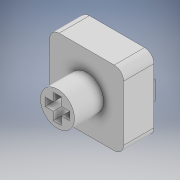
# Autodesk Inventor part: IPC ENTR key
Saved by Autodesk Inventor 2022 (Build 260153000, 153)
## iProperties
Created: 2021-12-31
Part Number: IPC ENTR key
Material: Generic
Document SubType Name: Modeling
Designer: solor
Density: 1 g/cm^3
Appearance: Default
Author: solor
Autodesk Inventor part; units mm, degrees
ref_plane "YZ Plane" through (0, 0, 0) normal (1, 0, 0) x (0, 1, 0)
ref_plane "XZ Plane" through (0, 0, 0) normal (0, 1, 0) x (-1, 0, 0)
sketch "Sketch1" plane through (0, 0, 0) normal (0, 0, 1) x (1, 0, 0)
  line L0 (14.6962, 12.74) -> (14.6962, 0) construction
  line L1 (10.61, 12.2) -> (1.53, 12.2)
  arc A0 (1.53, 12.2) -> (0, 10.67) centre (1.53, 10.67) ccw
  line L2 (0, 10.67) -> (0, 1.53)
  arc A1 (0, 1.53) -> (1.53, 0) centre (1.53, 1.53) ccw
  line L3 (1.53, 0) -> (10.61, 0)
  arc A2 (10.61, 0) -> (12.14, 1.53) centre (10.61, 1.53) ccw
  arc A3 (12.14, 10.67) -> (10.61, 12.2) centre (10.61, 10.67) ccw
  line L4 (12.14, 10.67) -> (12.14, 1.53)
  point P0 (0, 0)
  point P1 (0, 0)
  dimension "d10" = 12.74
  constraints: 10 end point, 8 point on circle, 4 centre point, 2 vertical, 1 point on line
  measures "d10" distance of L0.start L0.end
ref_plane "Work Plane1" through (0, 0, 5) normal (0, 0, 1) x (1, 0, 0)
sketch "Sketch2" plane through (0, 0, 5) normal (0, 0, 1) x (1, 0, 0)
  line L0 (10.88, 12.74) -> (1.8, 12.74) projected
  line L1 (10.88, 12.74) -> (1.8, 12.74) projected
  arc A0 (1.8, 12.74) -> (0, 10.94) centre (1.8, 10.94) ccw projected
  line L2 (0, 10.94) -> (0, 1.8) projected
  arc A1 (0, 1.8) -> (1.8, 0) centre (1.8, 1.8) ccw projected
  line L3 (1.8, 0) -> (10.88, 0) projected
  arc A2 (10.88, 0) -> (12.68, 1.8) centre (10.88, 1.8) ccw projected
  line L4 (12.68, 1.8) -> (12.68, 10.94) projected
  arc A3 (12.68, 10.94) -> (10.88, 12.74) centre (10.88, 10.94) ccw projected
  circle A4 centre (6.34, 6.37) radius 2.8
  line L5 (5.665, 8.395) -> (7.015, 8.395)
  line L6 (7.015, 4.345) -> (5.665, 4.345)
  line L7 (5.665, 4.345) -> (7.015, 8.395) construction
  line L8 (5.665, 8.395) -> (7.015, 4.345) construction
  line L9 (8.365, 5.695) -> (8.365, 7.045)
  line L10 (4.315, 7.045) -> (4.315, 5.695)
  line L11 (4.315, 5.695) -> (8.365, 7.045) construction
  line L12 (8.365, 5.695) -> (4.315, 7.045) construction
  line L13 (4.315, 5.695) -> (5.665, 5.695)
  line L14 (7.015, 5.695) -> (8.365, 5.695)
  line L15 (5.665, 4.345) -> (5.665, 5.695)
  line L16 (5.665, 7.045) -> (5.665, 8.395)
  line L17 (8.365, 7.045) -> (7.015, 7.045)
  line L18 (5.665, 7.045) -> (4.315, 7.045)
  line L19 (7.015, 8.395) -> (7.015, 7.045)
  line L20 (7.015, 5.695) -> (7.015, 4.345)
  point P0 (0, 0)
  dimension "d3" = 5.6
  dimension "d4" = 4.05
  dimension "d5" = 1.35
  dimension "d6" = 4.05
  dimension "d7" = 1.35
  constraints: 32 end point, 10 parallel, 8 perpendicular, 4 midpoint, 2 vertical, 1 centre point
  measures "d3" diameter of A4
  measures "d4" distance of L6.end L5.start
  measures "d5" distance of L5.start L5.end
  measures "d6" distance of L10.end L9.start
  measures "d7" distance of L9.end L9.start
extrude "Extrusion3" add sketch "Sketch1" along normal blind 5
sketch "Sketch3" plane through (0, 0, 5) normal (0, 0, 1) x (1, 0, 0)
  line L0 (10.61, 12.47) -> (1.53, 12.47)
  line L1 (10.61, 12.47) -> (1.53, 12.47)
  arc A0 (1.53, 12.47) -> (-0.27, 10.67) centre (1.53, 10.67) ccw
  line L2 (-0.27, 10.67) -> (-0.27, 1.53)
  arc A1 (-0.27, 1.53) -> (1.53, -0.27) centre (1.53, 1.53) ccw
  line L3 (1.53, -0.27) -> (10.61, -0.27)
  arc A2 (10.61, -0.27) -> (12.41, 1.53) centre (10.61, 1.53) ccw
  line L4 (12.41, 1.53) -> (12.41, 10.67)
  arc A3 (12.41, 10.67) -> (10.61, 12.47) centre (10.61, 10.67) ccw
  circle A4 centre (6.07, 6.1) radius 2.8
  line L5 (5.395, 8.125) -> (6.745, 8.125)
  line L6 (6.745, 4.075) -> (5.395, 4.075)
  line L7 (5.395, 4.075) -> (6.745, 8.125) construction
  line L8 (5.395, 8.125) -> (6.745, 4.075) construction
  line L9 (8.095, 5.425) -> (8.095, 6.775)
  line L10 (4.045, 6.775) -> (4.045, 5.425)
  line L11 (4.045, 5.425) -> (8.095, 6.775) construction
  line L12 (8.095, 5.425) -> (4.045, 6.775) construction
  line L13 (4.045, 5.425) -> (5.395, 5.425)
  line L14 (6.745, 5.425) -> (8.095, 5.425)
  line L15 (5.395, 4.075) -> (5.395, 5.425)
  line L16 (5.395, 6.775) -> (5.395, 8.125)
  line L17 (8.095, 6.775) -> (6.745, 6.775)
  line L18 (5.395, 6.775) -> (4.045, 6.775)
  line L19 (6.745, 8.125) -> (6.745, 6.775)
  line L20 (6.745, 5.425) -> (6.745, 4.075)
  line L21 (10.61, 12.2) -> (1.53, 12.2) projected
  line L22 (0, 10.67) -> (0, 1.53) projected
  point P0 (0, 0)
  point P1 (-0.27, -0.27)
  point P2 (6.07, 12.2)
  point P3 (0, 6.1)
  point P4 (6.07, 6.1)
  dimension "d14" = 5.6
  dimension "d15" = 4.05
  dimension "d16" = 1.35
  dimension "d17" = 4.05
  dimension "d18" = 1.35
  constraints: 42 end point, 10 parallel, 8 perpendicular, 8 point on circle, 6 midpoint, 5 centre point, 2 vertical
  measures "d14" diameter of A4
  measures "d15" distance of L6.end L5.start
  measures "d16" distance of L5.start L5.end
  measures "d17" distance of L10.end L9.start
  measures "d18" distance of L9.end L9.start
extrude "Extrusion4" add sketch "Sketch3" along normal blind 4.8 contours A4
sketch "Sketch4" plane through (0, 0, 0) normal (0, 0, -1) x (-1, 0, 0)
  line L0 (-13.9436, 0) -> (-13.9436, 2.266)
  line L1 (-15.5559, 0) -> (-15.5559, 6.84)
  line L2 (-1.53, 0) -> (-10.61, 0) projected
  line L3 (-11.7832, 7.625) -> (-0.3568, 7.625) construction
  line L4 (-0.3568, 7.625) -> (-0.3568, 4.575) construction
  line L5 (-0.3568, 4.575) -> (-11.7832, 4.575) construction
  line L6 (-11.7832, 4.575) -> (-11.7832, 7.625) construction
  line L7 (-11.4668, 4.575) -> (-11.4668, 7.625)
  line L8 (-11.4668, 7.625) -> (-9.4055, 7.625)
  line L9 (-9.4055, 7.625) -> (-9.4055, 7.0442)
  line L10 (-9.4055, 7.0442) -> (-10.7056, 7.0442)
  line L11 (-10.7056, 7.0442) -> (-10.7056, 6.5078)
  line L12 (-10.7056, 6.5078) -> (-9.5068, 6.5078)
  line L13 (-9.5068, 6.5078) -> (-9.5068, 5.927)
  line L14 (-9.5068, 5.927) -> (-10.7056, 5.927)
  line L15 (-10.7056, 5.927) -> (-10.7056, 5.1558)
  line L16 (-10.7056, 5.1558) -> (-9.4055, 5.1558)
  line L17 (-9.4055, 5.1558) -> (-9.4055, 4.575)
  line L18 (-9.4055, 4.575) -> (-11.4668, 4.575)
  line L19 (-6.2739, 4.575) -> (-7.0105, 4.575)
  line L20 (-7.0105, 4.575) -> (-8.187, 6.7006)
  line L21 (-8.187, 6.7006) -> (-8.187, 4.575)
  line L22 (-8.187, 4.575) -> (-8.8864, 4.575)
  line L23 (-8.8864, 4.575) -> (-8.8864, 7.625)
  line L24 (-8.8864, 7.625) -> (-7.9472, 7.625)
  line L25 (-7.9472, 7.625) -> (-6.9734, 5.8776)
  line L26 (-6.9734, 5.8776) -> (-6.9734, 7.625)
  line L27 (-6.9734, 7.625) -> (-6.2739, 7.625)
  line L28 (-6.2739, 7.625) -> (-6.2739, 4.575)
  line L29 (-5.0678, 4.575) -> (-5.0678, 7.0442)
  line L30 (-5.0678, 7.0442) -> (-5.9699, 7.0442)
  line L31 (-5.9699, 7.0442) -> (-5.9699, 7.625)
  line L32 (-5.9699, 7.625) -> (-3.3994, 7.625)
  line L33 (-3.3994, 7.625) -> (-3.3994, 7.0442)
  line L34 (-3.3994, 7.0442) -> (-4.3015, 7.0442)
  line L35 (-4.3015, 7.0442) -> (-4.3015, 4.575)
  line L36 (-4.3015, 4.575) -> (-5.0678, 4.575)
  line L37 (-0.2678, 4.575) -> (-1.1996, 4.575)
  line L38 (-1.1996, 4.575) -> (-2.0474, 5.6947)
  line L39 (-2.0474, 5.6947) -> (-2.3242, 5.6947)
  line L40 (-2.3242, 5.6947) -> (-2.3242, 4.575)
  line L41 (-2.3242, 4.575) -> (-3.0855, 4.575)
  line L42 (-3.0855, 4.575) -> (-3.0855, 7.625)
  line L43 (-3.0855, 7.625) -> (-1.8596, 7.625)
  spline S0 degree 2 poles (-1.8596, 7.625) (-1.605, 7.625) (-1.2293, 7.5607) (-1.0686, 7.4619) knots 0 0 0 1 2 2 2
  spline S1 degree 2 poles (-1.0686, 7.4619) (-0.9055, 7.3581) (-0.7127, 7.0343) (-0.7127, 6.7871) knots 0 0 0 1 2 2 2
  spline S2 degree 2 poles (-0.7127, 6.7871) (-0.7127, 6.4386) (-1.0291, 6.0011) (-1.2936, 5.8726) knots 0 0 0 1 2 2 2
  line L44 (-1.2936, 5.8726) -> (-0.2678, 4.575)
  spline S3 degree 2 poles (-1.4987, 6.6907) (-1.4987, 6.8069) (-1.5877, 6.9725) (-1.689, 7.017) knots 0 0 0 1 2 2 2
  spline S4 degree 2 poles (-1.689, 7.017) (-1.7607, 7.0466) (-1.9362, 7.0639) (-2.0672, 7.0639) knots 0 0 0 1 2 2 2
  line L45 (-2.0672, 7.0639) -> (-2.3242, 7.0639)
  line L46 (-2.3242, 7.0639) -> (-2.3242, 6.2434)
  line L47 (-2.3242, 6.2434) -> (-2.1043, 6.2434)
  spline S5 degree 2 poles (-2.1043, 6.2434) (-1.9461, 6.2434) (-1.7212, 6.2829) (-1.6445, 6.3447) knots 0 0 0 1 2 2 2
  spline S6 degree 2 poles (-1.6445, 6.3447) (-1.5704, 6.404) (-1.4987, 6.5622) (-1.4987, 6.6907) knots 0 0 0 1 2 2 2
  point P0 (0, 0)
  point P1 (-6.07, 0)
  point P2 (-6.07, 2.266)
  point P3 (-6.07, 6.84)
  point P4 (-6.07, 6.1)
  point P5 (-6.07, 4.575)
  point P6 (-0.3568, 6.1)
  point P7 (-6.07, 6.1)
  dimension "d21" = 2.266
  dimension "d22" = 6.84
  constraints: 4 end point, 3 midpoint, 2 vertical, 2 other
  measures "d21" distance of L0.start L0.end
  measures "d22" distance of L1.start L1.end
extrude "Extrusion5" add sketch "Sketch4" along normal blind 0.9
body "Solid2"
